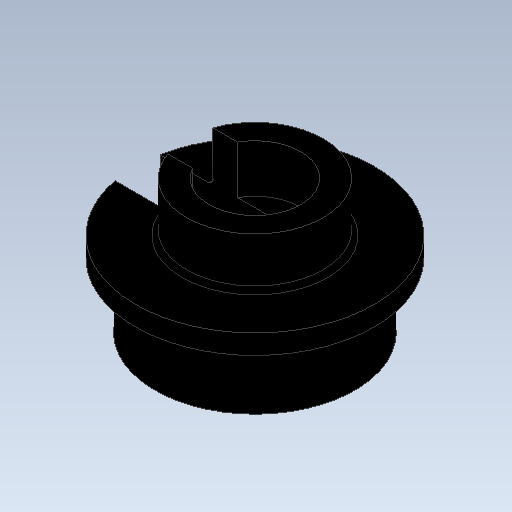
# Autodesk Inventor part: Pieza_Presion_resorte
Saved by Autodesk Inventor 2020 (Build 240168000, 168)
## iProperties
Created: 2019-09-21
Part Number: Pieza_Presion_resorte
Material: Plástico ABS
Document SubType Name: Modeling
Designer: axelj
Density: 1.06 g/cm^3
Appearance: Anodizado - Negro
Author: axelj
Autodesk Inventor part; units mm, degrees
ref_plane "YZ Plane" through (0, 0, 0) normal (1, 0, 0) x (0, 1, 0)
ref_plane "XZ Plane" through (0, 0, 0) normal (0, 1, 0) x (-1, 0, 0)
ref_plane "XY Plane" through (0, 0, 0) normal (0, 0, 1) x (1, 0, 0)
sketch "Boceto1" plane through (0, 0, 0) normal (0, 1, 0) x (-1, 0, 0)
  circle A0 centre (0, 0) radius 7.95
  dimension "d0" = 15.9
  constraints: 1 centre point, 1 coincident
  measures "d0" diameter of A0
extrude "Extrusión1" add sketch "Boceto1" along normal blind 1.3
sketch "Boceto2" plane through (0, 1.3, 0) normal (0, 1, 0) x (1, 0, 0)
  circle A0 centre (0, 0) radius 4.55
  dimension "d3" = 9.1
  constraints: 1 centre point, 1 coincident
  measures "d3" diameter of A0
extrude "Extrusión2" add sketch "Boceto2" along normal blind 3.3
sketch "Boceto3" plane through (0, 4.6, 0) normal (0, 1, 0) x (1, 0, 0)
  circle A0 centre (0, 0) radius 3.05
  dimension "d6" = 6.1
  constraints: 1 centre point, 1 coincident
  measures "d6" diameter of A0
extrude "Extrusión3" cut sketch "Boceto3" against normal blind 3.2
sketch "Boceto4" plane through (0, 1.4, 0) normal (0, 1, 0) x (1, 0, 0)
  arc A0 (0, -1.5) -> (0, 1.5) centre (0, 0) ccw
  line L0 (0, -1.5) -> (-7.8072, -1.5)
  circle A1 centre (0, 0) radius 7.95 projected
  line L1 (0, 1.5) -> (-7.8072, 1.5)
  arc A2 (-7.8072, 1.5) -> (-7.8072, -1.5) centre (0, 0) ccw
  dimension "d9" = 3
  constraints: 6 point on circle, 4 end point, 2 centre point, 2 coincident, 1 concentric, 1 horizontal, 1 parallel, 1 tangent
  measures "d9" diameter of A0
extrude "Extrusión4" cut sketch "Boceto4" along normal blind 3.2 and the other way blind 1.6 contours L0 A1 L1 A0 picked at (-2.6447, -0.1676)
fillet "Empalme1" radius 0.3 1 edges at (4.55, 1.3, 0)
sketch "Boceto5" plane through (0, 0, 0) normal (0, -1, 0) x (1, 0, 0)
  arc A0 (-6.4786, -1.5) -> (-6.4786, 1.5) centre (0, 0) ccw
  arc A1 (-5.5509, -1.5) -> (-5.5509, 1.5) centre (0, 0) ccw
  line L0 (-7.8072, 1.5) -> (0, 1.5) projected
  line L1 (-5.5509, 1.5) -> (-6.4786, 1.5)
  line L2 (-7.8072, -1.5) -> (-4.6122, -1.5) projected
  line L3 (-6.4786, -1.5) -> (-5.5509, -1.5)
  dimension "d15" = 13.3
  dimension "d16" = 11.5
  constraints: 4 end point, 4 point on circle, 4 point on line, 2 centre point, 2 coincident
  measures "d15" diameter of A0
  measures "d16" diameter of A1
extrude "Extrusión5" add sketch "Boceto5" along normal blind 4.3
